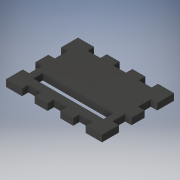
# Autodesk Inventor part: left
Saved by Autodesk Inventor 2019 (Build 230136000, 136)
## iProperties
Created: 2018-06-06
Part Number: left
Material: PBT Plastic Black
Document SubType Name: Modeling
Designer: stra92745
Density: 1.31 g/cm^3
Appearance: Smooth - White
Author: stra92745
Autodesk Inventor part; units mm, degrees
ref_plane "YZ Plane" through (0, 0, 0) normal (1, 0, 0) x (0, 1, 0)
ref_plane "XZ Plane" through (0, 0, 0) normal (0, 1, 0) x (-1, 0, 0)
ref_plane "XY Plane" through (0, 0, 0) normal (0, 0, 1) x (1, 0, 0)
sketch "Sketch1" plane through (0, 0, 0) normal (0, 1, 0) x (-1, 0, 0)
  line L0 (0, 0) -> (-60, 0)
  line L1 (-60, 0) -> (-60, -45)
  line L2 (-60, -45) -> (0, -45)
  line L3 (0, -45) -> (0, 0)
  line L4 (-8, -15) -> (-52, -15)
  line L5 (-52, -15) -> (-52, -9)
  line L6 (-52, -9) -> (-8, -9)
  line L7 (-8, -9) -> (-8, -15)
  dimension "d0" = 60
  dimension "d1" = 45
  dimension "d14" = 44
  dimension "d15" = 6
  dimension "d16" = 8
  dimension "d17" = 9
  constraints: 16 end point, 4 parallel, 2 horizontal, 2 perpendicular
  measures "d0" distance of L2.end L1.end
  measures "d1" distance of L1.end L0.end
  measures "d14" distance of L5.end L6.end
  measures "d15" distance of L4.end L5.end
  measures "d16" distance between parallel lines of L3 L7
  measures "d17" distance between parallel lines of L0 L6
extrude "Extrusion1" add sketch "Sketch1" along normal blind 4
sketch "Sketch2" plane through (0, 4, 0) normal (0, 1, 0) x (1, 0, 0)
  line L0 (0, 0) -> (60, 0) construction
  line L1 (60, 0) -> (60, 45) construction
  line L2 (60, 45) -> (0, 45) construction
  line L3 (0, 45) -> (0, 0) construction
  line L4 (4, 41) -> (56, 41) construction
  line L5 (56, 41) -> (56, 4) construction
  line L6 (56, 4) -> (4, 4) construction
  line L7 (4, 4) -> (4, 41) construction
  line L8 (60, 45) -> (0, 45) construction
  line L9 (30, 45) -> (30, 0) construction
  line L10 (0, 0) -> (60, 0) construction
  line L11 (0, 45) -> (0, 0) construction
  line L12 (0, 22.5) -> (60, 22.5) construction
  line L13 (60, 0) -> (60, 45) construction
  line L14 (0, 26.5) -> (4, 26.5)
  line L15 (0, 34.5) -> (4, 34.5)
  line L16 (10, 45) -> (10, 41)
  line L17 (10, 41) -> (18, 41)
  line L18 (18, 41) -> (18, 45)
  line L19 (18, 45) -> (10, 45)
  line L20 (26, 45) -> (26, 41)
  line L21 (26, 41) -> (30, 41)
  line L22 (26, 45) -> (30, 45)
  line L23 (0, 34.5) -> (0, 26.5)
  line L24 (4, 26.5) -> (4, 34.5)
  line L25 (60, 26.5) -> (56, 26.5)
  line L26 (60, 34.5) -> (56, 34.5)
  line L27 (50, 45) -> (50, 41)
  line L28 (50, 41) -> (42, 41)
  line L29 (42, 41) -> (42, 45)
  line L30 (42, 45) -> (50, 45)
  line L31 (34, 45) -> (34, 41)
  line L32 (34, 41) -> (30, 41)
  line L33 (34, 45) -> (30, 45)
  line L34 (60, 34.5) -> (60, 26.5)
  line L35 (56, 26.5) -> (56, 34.5)
  line L36 (60, 0) -> (0, 0) construction
  line L37 (4, 4) -> (56, 4) construction
  line L38 (60, 0) -> (0, 0) construction
  line L39 (0, 18.5) -> (4, 18.5)
  line L40 (0, 10.5) -> (4, 10.5)
  line L41 (10, 0) -> (10, 4)
  line L42 (10, 4) -> (18, 4)
  line L43 (18, 4) -> (18, 0)
  line L44 (18, 0) -> (10, 0)
  line L45 (26, 0) -> (26, 4)
  line L46 (26, 4) -> (30, 4)
  line L47 (26, 0) -> (30, 0)
  line L48 (0, 10.5) -> (0, 18.5)
  line L49 (4, 18.5) -> (4, 10.5)
  line L50 (34, 0) -> (34, 4)
  line L51 (34, 4) -> (30, 4)
  line L52 (34, 0) -> (30, 0)
  line L53 (42, 4) -> (42, 0)
  line L54 (50, 4) -> (42, 4)
  line L55 (42, 0) -> (50, 0)
  line L56 (50, 0) -> (50, 4)
  line L57 (56, 18.5) -> (56, 10.5)
  line L58 (60, 10.5) -> (56, 10.5)
  line L59 (60, 10.5) -> (60, 18.5)
  line L60 (60, 18.5) -> (56, 18.5)
  dimension "d4" = 4
  dimension "d7" = 8
  dimension "d8" = 8
  dimension "d9" = 4
  dimension "d10" = 8
  dimension "d11" = 4
  constraints: 106 end point, 31 symmetric about line, 16 point on line, 6 midpoint, 4 perpendicular, 3 collinear, 1 horizontal, 1 vertical, 3 other
  measures "d4" distance between parallel lines of L2 L4
  measures "d7" distance between parallel lines of L14 L15
  measures "d8" distance of L16.end L17.end
  measures "d9" distance of L20.end L21.end
  measures "d10" distance between parallel lines of L18 L20
  measures "d11" distance between parallel lines of L12 L14
extrude "Extrusion2" cut sketch "Sketch2" against normal up to surface (4 mm away)
body "Solid1"
